Autodesk Fusion 360 part; units mm, degrees
note: some values were not read from the file. Set by a fixed rule: which sketch regions a step uses.
(part 4 of 6)
  line L2804 (355, -75.3453) -> (353, -74.1906)
  line L2805 (391.5, -47.1906) -> (389.5, -48.3453)
  line L2806 (378.5, -84.3453) -> (378.5, -86.6547)
  line L2807 (389.5, -75.3453) -> (389.5, -77.6547)
  line L2808 (384, -75.3453) -> (384, -77.6547)
  line L2809 (369.5, -74.1906) -> (367.5, -75.3453)
  line L2810 (390.75, -79.5822) -> (388.75, -78.4275)
  line L2811 (389.5, -48.3453) -> (389.5, -50.6547)
  line L2812 (369.5, -74.1906) -> (367.5, -75.3453)
  line L2813 (352.25, -88.5822) -> (350.25, -87.4275)
  line L2814 (386, -78.8094) -> (388, -77.6547)
  line L2815 (377.75, -83.0463) -> (379.75, -81.8916)
  line L2816 (364, -78.8094) -> (366, -77.6547)
  line L2817 (377, -77.6547) -> (377, -75.3453)
  line L2818 (366.75, -74.0463) -> (368.75, -72.8916)
  line L2819 (388.75, -51.4275) -> (386.75, -52.5822)
  line L2820 (389.5, -77.6547) -> (391.5, -78.8094)
  line L2821 (390.75, -52.5822) -> (388.75, -51.4275)
  line L2822 (368.75, -79.5822) -> (366.75, -78.4275)
  line L2823 (364.75, -72.8916) -> (366.75, -74.0463)
  line L2824 (389.5, -75.3453) -> (389.5, -77.6547)
  line L2825 (366, -75.3453) -> (364, -74.1906)
  line L2826 (371.5, -48.3453) -> (369.5, -47.1906)
  line L2827 (367.5, -75.3453) -> (367.5, -77.6547)
  line L2828 (346.75, -81.8916) -> (346.75, -79.5822)
  line L2829 (377.75, -78.4275) -> (375.75, -79.5822)
  line L2830 (388, -75.3453) -> (386, -74.1906)
  line L2831 (364, -78.8094) -> (366, -77.6547)
  line L2832 (345.5, -84.3453) -> (345.5, -86.6547)
  line L2833 (384, -57.3453) -> (384, -59.6547)
  line L2834 (390.75, -79.5822) -> (388.75, -78.4275)
  line L2835 (375.75, -79.5822) -> (375.75, -81.8916)
  line L2836 (384, -77.6547) -> (386, -78.8094)
  line L2837 (366, -77.6547) -> (366, -75.3453)
  line L2838 (348.25, -81.8916) -> (350.25, -83.0463)
  line L2839 (367.5, -57.3453) -> (367.5, -59.6547)
  line L2840 (379.75, -79.5822) -> (377.75, -78.4275)
  line L2841 (355.75, -56.0463) -> (357.75, -54.8916)
  line L2842 (348.25, -53.9293) -> (348.25, -54.8916)
  line L2843 (377.75, -47.0463) -> (379.75, -45.8916)
  line L2844 (384, -57.3453) -> (384, -59.6547)
  line L2845 (380.5, -74.1906) -> (378.5, -75.3453)
  line L2846 (349.5, -84.3453) -> (347.5, -83.1906)
  line L2847 (389.5, -57.3453) -> (389.5, -59.6547)
  line L2848 (380.5, -78.8094) -> (382.5, -77.6547)
  line L2849 (355, -59.6547) -> (355, -57.3453)
  line L2850 (381.25, -79.5822) -> (381.25, -81.8916)
  line L2851 (348.25, -79.5822) -> (348.25, -81.8916)
  line L2852 (391.5, -56.1906) -> (389.5, -57.3453)
  line L2853 (348.25, -79.5822) -> (348.25, -81.8916)
  line L2854 (368.75, -79.5822) -> (366.75, -78.4275)
  line L2855 (386.75, -43.5822) -> (386.75, -45.8916)
  line L2856 (367.5, -75.3453) -> (367.5, -77.6547)
  line L2857 (353, -83.1906) -> (351, -84.3453)
  line L2858 (380.5, -78.8094) -> (382.5, -77.6547)
  line L2859 (350.25, -87.4275) -> (348.25, -88.5822)
  line L2860 (386, -60.8094) -> (388, -59.6547)
  line L2861 (377.75, -78.4275) -> (375.75, -79.5822)
  line L2862 (357.75, -61.5822) -> (355.75, -60.4275)
  line L2863 (380.5, -51.8094) -> (382.5, -50.6547)
  line L2864 (378.5, -77.6547) -> (380.5, -78.8094)
  line L2865 (346.75, -81.8916) -> (346.75, -79.5822)
  line L2866 (388, -59.6547) -> (388, -57.3453)
  line L2867 (381.25, -79.5822) -> (381.25, -81.8916)
  line L2868 (375.75, -79.5822) -> (375.75, -81.8916)
  line L2869 (386, -56.1906) -> (384, -57.3453)
  line L2870 (367.5, -77.6547) -> (369.5, -78.8094)
  line L2871 (349.5, -84.3453) -> (347.5, -83.1906)
  line L2872 (364.75, -72.8916) -> (366.75, -74.0463)
  line L2873 (349.5, -86.6547) -> (349.5, -84.3453)
  line L2874 (380.5, -47.1906) -> (378.5, -48.3453)
  line L2875 (392.25, -61.5822) -> (392.25, -63.8916)
  line L2876 (390.75, -45.8916) -> (390.75, -45.244)
  line L2877 (357.75, -61.5822) -> (355.75, -60.4275)
  line L2878 (385.25, -45.8916) -> (385.25, -43.5822)
  line L2879 (366.75, -78.4275) -> (364.75, -79.5822)
  line L2880 (367.5, -77.6547) -> (369.5, -78.8094)
  line L2881 (382.5, -77.6547) -> (382.5, -75.3453)
  line L2882 (375.75, -43.5822) -> (375.75, -45.8916)
  line L2883 (353.75, -54.8916) -> (355.75, -56.0463)
  line L2884 (366, -75.3453) -> (364, -74.1906)
  line L2885 (346.75, -88.5822) -> (344.75, -87.4275)
  line L2886 (344.75, -83.0463) -> (346.75, -81.8916)
  line L2887 (356.5, -59.6547) -> (358.5, -60.8094)
  line L2888 (390.75, -45.8916) -> (390.75, -45.244)
  line L2889 (366, -59.6547) -> (366, -57.3453)
  line L2890 (382.5, -75.3453) -> (380.5, -74.1906)
  line L2891 (382.5, -75.3453) -> (380.5, -74.1906)
  line L2892 (386, -56.1906) -> (384, -57.3453)
  line L2893 (384, -59.6547) -> (386, -60.8094)
  line L2894 (351, -86.6547) -> (353, -87.8094)
  line L2895 (382.5, -50.6547) -> (382.5, -48.3453)
  line L2896 (358.5, -60.8094) -> (360.5, -59.6547)
  line L2897 (367.5, -57.3453) -> (367.5, -59.6547)
  line L2898 (379.75, -79.5822) -> (377.75, -78.4275)
  line L2899 (351, -84.3453) -> (351, -86.6547)
  line L2900 (355.75, -60.4275) -> (353.75, -61.5822)
  line L2901 (388.75, -60.4275) -> (386.75, -61.5822)
  line L2902 (352.25, -81.8916) -> (352.25, -79.5822)
  line L2903 (377, -77.6547) -> (377, -75.3453)
  arc A93 (390.75, -45.244) -> (386.8045, -43.5507) centre (375, -76.5) ccw
  line L2904 (386.8045, -43.5507) -> (386.75, -43.5822)
  line L2905 (351, -84.3453) -> (351, -86.6547)
  line L2906 (347.5, -83.1906) -> (345.5, -84.3453)
  line L2907 (349.5, -86.6547) -> (349.5, -84.3453)
  line L2908 (366, -59.6547) -> (366, -57.3453)
  line L2909 (377, -41.6547) -> (377, -41.5572)
  line L2910 (355.75, -60.4275) -> (353.75, -61.5822)
  line L2911 (345.5, -86.6547) -> (347.5, -87.8094)
  line L2912 (379.75, -81.8916) -> (379.75, -79.5822)
  line L2913 (351, -86.6547) -> (353, -87.8094)
  line L2914 (361.25, -60.4275) -> (359.25, -61.5822)
  line L2915 (385.25, -63.8916) -> (385.25, -61.5822)
  line L2916 (386.75, -54.8916) -> (388.75, -56.0463)
  line L2917 (344.75, -83.0463) -> (346.75, -81.8916)
  line L2918 (378.5, -50.6547) -> (380.5, -51.8094)
  line L2919 (378.5, -75.3453) -> (378.5, -77.6547)
  line L2920 (379.75, -52.5822) -> (377.75, -51.4275)
  line L2921 (359.25, -54.8916) -> (361.25, -56.0463)
  line L2922 (377.75, -47.0463) -> (379.75, -45.8916)
  line L2923 (367.5, -66.3453) -> (367.5, -68.6547)
  line L2924 (379.75, -81.8916) -> (379.75, -79.5822)
  line L2925 (352.25, -81.8916) -> (352.25, -79.5822)
  line L2926 (386.75, -54.8916) -> (388.75, -56.0463)
  line L2927 (386, -60.8094) -> (388, -59.6547)
  line L2928 (350.25, -83.0463) -> (352.25, -81.8916)
  line L2929 (360.5, -57.3453) -> (358.5, -56.1906)
  line L2930 (360.5, -57.3453) -> (358.5, -56.1906)
  line L2931 (378.5, -75.3453) -> (378.5, -77.6547)
  line L2932 (378.5, -48.3453) -> (378.5, -50.6547)
  line L2933 (378.5, -77.6547) -> (380.5, -78.8094)
  line L2934 (350.25, -87.4275) -> (348.25, -88.5822)
  line L2935 (355, -59.6547) -> (355, -57.3453)
  line L2936 (382.5, -50.6547) -> (382.5, -48.3453)
  line L2937 (391.5, -56.1906) -> (389.5, -57.3453)
  line L2938 (362, -57.3453) -> (362, -59.6547)
  line L2939 (388.75, -56.0463) -> (390.75, -54.8916)
  line L2940 (345.5, -86.6547) -> (347.5, -87.8094)
  line L2941 (379.75, -43.5822) -> (377.75, -42.4275)
  line L2942 (388.75, -60.4275) -> (386.75, -61.5822)
  line L2943 (347.5, -83.1906) -> (345.5, -84.3453)
  line L2944 (362, -57.3453) -> (362, -59.6547)
  line L2945 (377, -50.6547) -> (377, -48.3453)
  line L2946 (388, -57.3453) -> (386, -56.1906)
  line L2947 (381.25, -61.5822) -> (381.25, -63.8916)
  line L2948 (366, -66.3453) -> (364, -65.1906)
  line L2949 (382.5, -77.6547) -> (382.5, -75.3453)
  line L2950 (378.5, -48.3453) -> (378.5, -50.6547)
  line L2951 (388, -57.3453) -> (386, -56.1906)
  line L2952 (377, -50.6547) -> (377, -48.3453)
  line L2953 (358.5, -60.8094) -> (360.5, -59.6547)
  line L2954 (358.5, -56.1906) -> (356.5, -57.3453)
  line L2955 (389.5, -59.6547) -> (391.5, -60.8094)
  line L2956 (378.5, -50.6547) -> (380.5, -51.8094)
  line L2957 (382.5, -48.3453) -> (380.5, -47.1906)
  line L2958 (389.5, -59.6547) -> (391.5, -60.8094)
  line L2959 (350.25, -83.0463) -> (352.25, -81.8916)
  line L2960 (366.75, -69.4275) -> (364.75, -70.5822)
  line L2961 (358.5, -56.1906) -> (356.5, -57.3453)
  line L2962 (379.75, -52.5822) -> (377.75, -51.4275)
  line L2963 (388, -59.6547) -> (388, -57.3453)
  line L2964 (363.25, -63.8916) -> (363.25, -61.5822)
  line L2965 (351, -77.6547) -> (353, -78.8094)
  line L2966 (382.5, -48.3453) -> (380.5, -47.1906)
  line L2967 (359.25, -54.8916) -> (361.25, -56.0463)
  line L2968 (378.5436, -41.6798) -> (380.5, -42.8094)
  arc A94 (381.6602, -42.1395) -> (378.5436, -41.6798) centre (375, -76.5) ccw
  line L2969 (378.5436, -41.6798) -> (380.5, -42.8094)
  line L2970 (349.5, -77.6547) -> (349.5, -75.3453)
  line L2971 (377.75, -51.4275) -> (375.75, -52.5822)
  line L2972 (369.5, -56.1906) -> (367.5, -57.3453)
  line L2973 (380.5, -42.8094) -> (381.6602, -42.1395)
  line L2974 (375.75, -45.8916) -> (377.75, -47.0463)
  line L2975 (364.75, -54.8916) -> (366.75, -56.0463)
  line L2976 (367.5, -59.6547) -> (369.5, -60.8094)
  line L2977 (345.5, -84.3453) -> (345.5, -86.6547)
  line L2978 (347.5, -87.8094) -> (349.5, -86.6547)
  line L2979 (353.75, -54.8916) -> (355.75, -56.0463)
  line L2980 (375.75, -45.8916) -> (377.75, -47.0463)
  line L2981 (380.5, -47.1906) -> (378.5, -48.3453)
  line L2982 (353, -83.1906) -> (351, -84.3453)
  line L2983 (364, -60.8094) -> (366, -59.6547)
  line L2984 (356.5, -59.6547) -> (358.5, -60.8094)
  line L2985 (366.75, -51.4275) -> (364.75, -52.5822)
  line L2986 (368.75, -63.8916) -> (368.75, -61.5822)
  line L2987 (368.75, -63.8916) -> (368.75, -61.5822)
  line L2988 (366.75, -56.0463) -> (368.75, -54.8916)
  line L2989 (368.75, -61.5822) -> (366.75, -60.4275)
  line L2990 (353, -74.1906) -> (351, -75.3453)
  line L2991 (380.5, -51.8094) -> (382.5, -50.6547)
  line L2992 (360.5, -59.6547) -> (360.5, -57.3453)
  line L2993 (369.5, -65.1906) -> (367.5, -66.3453)
  line L2994 (348.25, -81.8916) -> (350.25, -83.0463)
  line L2995 (355.75, -56.0463) -> (357.75, -54.8916)
  line L2996 (390.75, -61.5822) -> (388.75, -60.4275)
  line L2997 (345.5, -75.3453) -> (345.5, -77.6547)
  line L2998 (367.5, -68.6547) -> (369.5, -69.8094)
  line L2999 (377.75, -42.4275) -> (375.75, -43.5822)
  line L3000 (368.75, -70.5822) -> (366.75, -69.4275)
  line L3001 (366, -57.3453) -> (364, -56.1906)
  line L3002 (390.75, -61.5822) -> (388.75, -60.4275)
  line L3003 (384, -59.6547) -> (386, -60.8094)
  line L3004 (346.75, -88.5822) -> (344.75, -87.4275)
  line L3005 (366.75, -56.0463) -> (368.75, -54.8916)
  line L3006 (350.25, -74.0463) -> (352.25, -72.8916)
  line L3007 (356.5, -57.3453) -> (356.5, -59.6547)
  arc A95 (383.427, -42.5296) -> (383.1782, -42.4689) centre (375, -76.5) ccw
  line L3008 (366, -66.3453) -> (364, -65.1906)
  line L3009 (377.75, -51.4275) -> (375.75, -52.5822)
  line L3010 (352.25, -79.5822) -> (350.25, -78.4275)
  line L3011 (345.5, -77.6547) -> (347.5, -78.8094)
  line L3012 (361.25, -60.4275) -> (359.25, -61.5822)
  line L3013 (352.25, -79.5822) -> (350.25, -78.4275)
  line L3014 (352.25, -88.5822) -> (350.25, -87.4275)
  line L3015 (369.5, -56.1906) -> (367.5, -57.3453)
  line L3016 (360.5, -59.6547) -> (360.5, -57.3453)
  line L3017 (388.75, -56.0463) -> (390.75, -54.8916)
  line L3018 (364.75, -70.5822) -> (364.75, -72.8916)
  line L3019 (385.25, -52.5822) -> (383.25, -51.4275)
  line L3020 (349.5, -77.6547) -> (349.5, -75.3453)
  line L3021 (364, -51.8094) -> (366, -50.6547)
  line L3022 (366.75, -65.0463) -> (368.75, -63.8916)
  line L3023 (347.5, -74.1906) -> (345.5, -75.3453)
  line L3024 (364.75, -52.5822) -> (364.75, -54.8916)
  line L3025 (379.75, -43.5822) -> (377.75, -42.4275)
  line L3026 (368.75, -54.8916) -> (368.75, -52.5822)
  line L3027 (380.5, -56.1906) -> (378.5, -57.3453)
  line L3028 (345.5, -75.3453) -> (345.5, -77.6547)
  line L3029 (367.5, -59.6547) -> (369.5, -60.8094)
  line L3030 (347.5, -74.1906) -> (345.5, -75.3453)
  line L3031 (385.25, -52.5822) -> (383.25, -51.4275)
  line L3032 (366, -57.3453) -> (364, -56.1906)
  line L3033 (381.25, -45.8916) -> (383.25, -47.0463)
  line L3034 (357.75, -54.8916) -> (357.75, -52.5822)
  line L3035 (357.75, -63.8916) -> (357.75, -61.5822)
  line L3036 (363.25, -54.8916) -> (363.25, -52.5822)
  line L3037 (383.1782, -42.4689) -> (381.25, -43.5822)
  line L3038 (383.25, -47.0463) -> (385.25, -45.8916)
  line L3039 (346.75, -79.5822) -> (344.75, -78.4275)
  line L3040 (383.25, -51.4275) -> (381.25, -52.5822)
  line L3041 (367.5, -50.6547) -> (369.5, -51.8094)
  line L3042 (351, -77.6547) -> (353, -78.8094)
  line L3043 (369.5, -65.1906) -> (367.5, -66.3453)
  line L3044 (366.75, -65.0463) -> (368.75, -63.8916)
  line L3045 (368.75, -52.5822) -> (366.75, -51.4275)
  line L3046 (380.5, -60.8094) -> (382.5, -59.6547)
  line L3047 (377.75, -42.4275) -> (375.75, -43.5822)
  line L3048 (367.5, -68.6547) -> (369.5, -69.8094)
  line L3049 (347.5, -78.8094) -> (349.5, -77.6547)
  arc A96 (390.75, -45.244) -> (386.8045, -43.5507) centre (375, -76.5) ccw
  line L3050 (344.75, -74.0463) -> (346.75, -72.8916)
  line L3051 (347.5, -78.8094) -> (349.5, -77.6547)
  line L3052 (363.25, -54.8916) -> (363.25, -52.5822)
  line L3053 (364.75, -63.8916) -> (366.75, -65.0463)
  line L3054 (359.25, -61.5822) -> (359.25, -63.8916)
  line L3055 (359.25, -61.5822) -> (359.25, -63.8916)
  line L3056 (350.25, -78.4275) -> (348.25, -79.5822)
  line L3057 (353.75, -61.5822) -> (353.75, -63.8916)
  line L3058 (385.25, -43.5822) -> (383.427, -42.5296)
  line L3059 (356.5, -57.3453) -> (356.5, -59.6547)
  line L3060 (377.75, -56.0463) -> (379.75, -54.8916)
  line L3061 (359.25, -52.5822) -> (359.25, -54.8916)
  line L3062 (383.25, -51.4275) -> (381.25, -52.5822)
  line L3063 (349.5, -75.3453) -> (347.5, -74.1906)
  line L3064 (363.25, -72.8916) -> (363.25, -70.5822)
  line L3065 (364.75, -61.5822) -> (364.75, -63.8916)
  line L3066 (350.25, -78.4275) -> (348.25, -79.5822)
  line L3067 (381.25, -61.5822) -> (381.25, -63.8916)
  line L3068 (364, -69.8094) -> (366, -68.6547)
  line L3069 (344.75, -74.0463) -> (346.75, -72.8916)
  line L3070 (366.75, -69.4275) -> (364.75, -70.5822)
  line L3071 (364.75, -52.5822) -> (364.75, -54.8916)
  line L3072 (377, -41.6547) -> (377, -41.5572)
  line L3073 (385.25, -43.5822) -> (383.427, -42.5296)
  line L3074 (383.1782, -42.4689) -> (381.25, -43.5822)
  line L3075 (367.5, -48.3453) -> (367.5, -50.6547)
  line L3076 (383.25, -47.0463) -> (385.25, -45.8916)
  line L3077 (353.75, -61.5822) -> (353.75, -63.8916)
  arc A97 (381.6602, -42.1395) -> (378.5436, -41.6798) centre (375, -76.5) ccw
  line L3078 (366.75, -51.4275) -> (364.75, -52.5822)
  line L3079 (381.25, -45.8916) -> (383.25, -47.0463)
  line L3080 (357.75, -63.8916) -> (357.75, -61.5822)
  line L3081 (366.75, -60.4275) -> (364.75, -61.5822)
  line L3082 (348.25, -72.8916) -> (350.25, -74.0463)
  line L3083 (386.8045, -43.5507) -> (386.75, -43.5822)
  line L3084 (368.75, -52.5822) -> (366.75, -51.4275)
  line L3085 (377, -59.6547) -> (377, -57.3453)
  line L3086 (368.75, -54.8916) -> (368.75, -52.5822)
  line L3087 (375.75, -54.8916) -> (377.75, -56.0463)
  line L3088 (346.75, -70.5822) -> (344.75, -69.4275)
  line L3089 (367.5, -48.3453) -> (367.5, -50.6547)
  line L3090 (364.75, -43.5822) -> (364.75, -45.8916)
  line L3091 (363.25, -63.8916) -> (363.25, -61.5822)
  line L3092 (350.25, -74.0463) -> (352.25, -72.8916)
  line L3093 (355, -57.3453) -> (353, -56.1906)
  line L3094 (377.75, -60.4275) -> (375.75, -61.5822)
  line L3095 (364.75, -54.8916) -> (366.75, -56.0463)
  line L3096 (355, -57.3453) -> (353, -56.1906)
  line L3097 (368.75, -72.8916) -> (368.75, -70.5822)
  line L3098 (390.75, -63.8916) -> (390.75, -61.5822)
  line L3099 (366, -50.6547) -> (366, -48.3453)
  line L3100 (378.5, -57.3453) -> (378.5, -59.6547)
  line L3101 (364.75, -61.5822) -> (364.75, -63.8916)
  line L3102 (348.25, -72.8916) -> (350.25, -74.0463)
  line L3103 (353, -74.1906) -> (351, -75.3453)
  line L3104 (353, -60.8094) -> (355, -59.6547)
  line L3105 (351, -75.3453) -> (351, -77.6547)
  line L3106 (355, -66.3453) -> (353, -65.1906)
  line L3107 (368.75, -70.5822) -> (366.75, -69.4275)
  line L3108 (351, -75.3453) -> (351, -77.6547)
  line L3109 (377.75, -60.4275) -> (375.75, -61.5822)
  line L3110 (345.5, -77.6547) -> (347.5, -78.8094)
  line L3111 (359.25, -45.244) -> (359.25, -45.8916)
  line L3112 (366, -68.6547) -> (366, -66.3453)
  line L3113 (380.5, -60.8094) -> (382.5, -59.6547)
  line L3114 (348.25, -63.8916) -> (350.25, -65.0463)
  line L3115 (359.25, -45.244) -> (359.25, -45.8916)
  line L3116 (377, -59.6547) -> (377, -57.3453)
  line L3117 (380.5, -42.8094) -> (381.6602, -42.1395)
  line L3118 (368.75, -45.8916) -> (368.75, -43.5822)
  line L3119 (382.5, -57.3453) -> (380.5, -56.1906)
  line L3120 (346.75, -79.5822) -> (344.75, -78.4275)
  line L3121 (383.25, -56.0463) -> (385.25, -54.8916)
  line L3122 (353, -69.8094) -> (355, -68.6547)
  line L3123 (377.75, -56.0463) -> (379.75, -54.8916)
  line L3124 (364, -60.8094) -> (366, -59.6547)
  line L3125 (382.5, -59.6547) -> (382.5, -57.3453)
  line L3126 (366, -50.6547) -> (366, -48.3453)
  line L3127 (366.75, -60.4275) -> (364.75, -61.5822)
  line L3128 (375.75, -61.5822) -> (375.75, -63.8916)
  line L3129 (364.75, -63.8916) -> (366.75, -65.0463)
  line L3130 (368.3398, -42.1395) -> (369.5, -42.8094)
  line L3131 (364, -51.8094) -> (366, -50.6547)
  line L3132 (368.75, -61.5822) -> (366.75, -60.4275)
  line L3133 (352.25, -70.5822) -> (350.25, -69.4275)
  line L3134 (386.75, -61.5822) -> (386.75, -63.8916)
  line L3135 (367.5, -66.3453) -> (367.5, -68.6547)
  line L3136 (367.5, -50.6547) -> (369.5, -51.8094)
  line L3137 (364, -69.8094) -> (366, -68.6547)
  line L3138 (353, -60.8094) -> (355, -59.6547)
  line L3139 (379.75, -61.5822) -> (377.75, -60.4275)
  line L3140 (366, -68.6547) -> (366, -66.3453)
  line L3141 (382.5, -59.6547) -> (382.5, -57.3453)
  line L3142 (349.5, -75.3453) -> (347.5, -74.1906)
  line L3143 (385.25, -63.8916) -> (385.25, -61.5822)
  line L3144 (363.25, -43.5822) -> (363.1955, -43.5507)
  line L3145 (356.5, -50.6547) -> (358.5, -51.8094)
  line L3146 (379.75, -61.5822) -> (377.75, -60.4275)
  line L3147 (363.25, -72.8916) -> (363.25, -70.5822)
  line L3148 (368.75, -72.8916) -> (368.75, -70.5822)
  arc A98 (350.4572, -51.5471) -> (348.25, -53.9293) centre (375, -76.5) ccw
  line L3149 (357.75, -52.5822) -> (355.75, -51.4275)
  line L3150 (351, -66.3453) -> (351, -68.6547)
  line L3151 (385.25, -61.5822) -> (383.25, -60.4275)
  line L3152 (382.5, -57.3453) -> (380.5, -56.1906)
  line L3153 (356.5, -48.3453) -> (356.5, -50.6547)
  line L3154 (378.5, -57.3453) -> (378.5, -59.6547)
  line L3155 (355, -48.3453) -> (354.558, -48.0901)
  line L3156 (364.75, -70.5822) -> (364.75, -72.8916)
  line L3157 (353, -65.1906) -> (351, -66.3453)
  line L3158 (361.25, -51.4275) -> (359.25, -52.5822)
  line L3159 (405.25, -83.0463) -> (407.25, -81.8916)
  line L3160 (409.917, -78.9084) -> (408.75, -79.5822)
  line L3161 (405.25, -78.4275) -> (403.25, -79.5822)
  line L3162 (403.25, -79.5822) -> (403.25, -81.8916)
  line L3163 (408, -78.8094) -> (409.9806, -77.6659)
  line L3164 (409.211, -83.8898) -> (408, -83.1906)
  line L3165 (407.25, -81.8916) -> (407.25, -79.5822)
  line L3166 (405.25, -78.4275) -> (403.25, -79.5822)
  line L3167 (407.25, -79.5822) -> (405.25, -78.4275)
  arc A99 (409.5109, -82.3309) -> (409.917, -78.9084) centre (375, -76.5) ccw
  line L3168 (408, -83.1906) -> (406, -84.3453)
  line L3169 (407.25, -79.5822) -> (405.25, -78.4275)
  line L3170 (408, -78.8094) -> (409.9806, -77.6659)
  line L3171 (407.25, -72.8916) -> (407.25, -70.5822)
  line L3172 (375, -51.8094) -> (377, -50.6547)
  line L3173 (407.25, -70.5822) -> (405.25, -69.4275)
  line L3174 (404.5, -77.6547) -> (404.5, -75.3453)
  line L3175 (405.25, -74.0463) -> (407.25, -72.8916)
  line L3176 (409.4268, -70.1914) -> (408.75, -70.5822)
  line L3177 (408, -74.1906) -> (406, -75.3453)
  line L3178 (403.25, -70.5822) -> (403.25, -72.8916)
  line L3179 (406, -68.6547) -> (408, -69.8094)
  arc A100 (409.8747, -73.5409) -> (409.4268, -70.1914) centre (375, -76.5) ccw
  line L3180 (405.25, -69.4275) -> (403.25, -70.5822)
  line L3181 (408.75, -70.5822) -> (408.75, -72.8916)
  line L3182 (407.25, -72.8916) -> (407.25, -70.5822)
  line L3183 (408.75, -72.8916) -> (409.8747, -73.5409)
  line L3184 (407.25, -70.5822) -> (405.25, -69.4275)
  line L3185 (405.25, -74.0463) -> (407.25, -72.8916)
  line L3186 (403.25, -70.5822) -> (403.25, -72.8916)
  line L3187 (408, -74.1906) -> (406, -75.3453)
  line L3188 (408.75, -70.5822) -> (408.75, -72.8916)
  line L3189 (403.25, -72.8916) -> (405.25, -74.0463)
  line L3190 (409.4268, -70.1914) -> (408.75, -70.5822)
  arc A101 (410, -76.5) -> (409.9806, -75.3341) centre (375, -76.5) ccw
  arc A102 (410, -76.5) -> (409.9806, -75.3341) centre (375, -76.5) ccw
  line L3191 (403.25, -72.8916) -> (405.25, -74.0463)
  line L3192 (409.9806, -75.3341) -> (408, -74.1906)
  line L3193 (409.9806, -75.3341) -> (408, -74.1906)
  line L3194 (408.75, -72.8916) -> (409.8747, -73.5409)
  line L3195 (405.25, -69.4275) -> (403.25, -70.5822)
  arc A103 (409.8747, -73.5409) -> (409.4268, -70.1914) centre (375, -76.5) ccw
  line L3196 (408, -69.8094) -> (409.211, -69.1102)
  line L3197 (406, -77.6547) -> (408, -78.8094)
  arc A104 (409.9806, -77.6659) -> (410, -76.5) centre (375, -76.5) ccw
  line L3198 (406, -77.6547) -> (408, -78.8094)
  line L3199 (406, -75.3453) -> (406, -77.6547)
  line L3200 (406, -68.6547) -> (408, -69.8094)
  line L3201 (406, -75.3453) -> (406, -77.6547)
  line L3202 (404.5, -77.6547) -> (404.5, -75.3453)
  line L3203 (408, -69.8094) -> (409.211, -69.1102)
  arc A105 (409.9806, -77.6659) -> (410, -76.5) centre (375, -76.5) ccw
  arc A106 (392.25, -106.9539) -> (394.4942, -105.5685) centre (375, -76.5) ccw
  line L3204 (394.4942, -105.5685) -> (394.25, -105.4275)
  line L3205 (394.25, -105.4275) -> (392.25, -106.5822)
  arc A107 (392.25, -106.9539) -> (394.4942, -105.5685) centre (375, -76.5) ccw
  line L3206 (394.25, -105.4275) -> (392.25, -106.5822)
  line L3207 (394.4942, -105.5685) -> (394.25, -105.4275)
  line L3208 (386.75, -99.8916) -> (388.75, -101.0463)
  line L3209 (399.5428, -51.5471) -> (397.75, -52.5822)
  line L3210 (381.25, -88.5822) -> (381.25, -90.8916)
  line L3211 (362, -77.6547) -> (364, -78.8094)
  line L3212 (396.25, -63.8916) -> (396.25, -61.5822)
  line L3213 (368.75, -81.8916) -> (368.75, -79.5822)
  line L3214 (371.5, -68.6547) -> (371.5, -66.3453)
  line L3215 (388, -95.6547) -> (388, -93.3453)
  line L3216 (399, -66.3453) -> (397, -65.1906)
  line L3217 (386, -96.8094) -> (388, -95.6547)
  line L3218 (397, -51.8094) -> (398.7552, -50.7961)
  arc A108 (398.7552, -50.7961) -> (395.442, -48.0901) centre (375, -76.5) ccw
  line L3219 (372.25, -96.4275) -> (370.25, -97.5822)
  line L3220 (386, -92.1906) -> (384, -93.3453)
  line L3221 (386.75, -99.8916) -> (388.75, -101.0463)
  line L3222 (372.25, -69.4275) -> (370.25, -70.5822)
  line L3223 (392.25, -97.5822) -> (392.25, -99.8916)
  line L3224 (399.5428, -51.5471) -> (397.75, -52.5822)
  line L3225 (393.5, -50.6547) -> (393.5, -48.3453)
  line L3226 (375, -101.1906) -> (373, -102.3453)
  line L3227 (372.25, -60.4275) -> (370.25, -61.5822)
  line L3228 (371.5, -68.6547) -> (371.5, -66.3453)
  line L3229 (374.25, -97.5822) -> (372.25, -96.4275)
  line L3230 (395.442, -48.0901) -> (395, -48.3453)
  line L3231 (395, -48.3453) -> (395, -50.6547)
  line L3232 (396.25, -63.8916) -> (396.25, -61.5822)
  line L3233 (389.5, -93.3453) -> (389.5, -95.6547)
  line L3234 (390.75, -97.5822) -> (388.75, -96.4275)
  line L3235 (401.75, -61.5822) -> (399.75, -60.4275)
  line L3236 (390.75, -54.8916) -> (390.75, -52.5822)
  line L3237 (395.442, -48.0901) -> (395, -48.3453)
  line L3238 (370.25, -63.8916) -> (372.25, -65.0463)
  line L3239 (392.25, -88.5822) -> (392.25, -90.8916)
  line L3240 (402.5, -60.8094) -> (404.5, -59.6547)
  line L3241 (370.25, -99.8916) -> (372.25, -101.0463)
  line L3242 (399, -66.3453) -> (397, -65.1906)
  line L3243 (395, -48.3453) -> (395, -50.6547)
  line L3244 (389.5, -95.6547) -> (391.5, -96.8094)
  line L3245 (372.25, -92.0463) -> (374.25, -90.8916)
  line L3246 (401.75, -61.5822) -> (399.75, -60.4275)
  line L3247 (353.75, -70.5822) -> (353.75, -72.8916)
  line L3248 (370.25, -97.5822) -> (370.25, -99.8916)
  line L3249 (396.25, -52.5822) -> (394.25, -51.4275)
  line L3250 (394.25, -65.0463) -> (396.25, -63.8916)
  line L3251 (372.25, -96.4275) -> (370.25, -97.5822)
  line L3252 (397.75, -63.8916) -> (399.75, -65.0463)
  line L3253 (395, -59.6547) -> (397, -60.8094)
  line L3254 (375, -92.1906) -> (373, -93.3453)
  line L3255 (404.1665, -57.1527) -> (402.5, -56.1906)
  line L3256 (373, -59.6547) -> (375, -60.8094)
  line L3257 (384, -95.6547) -> (386, -96.8094)
  line L3258 (375, -65.1906) -> (373, -66.3453)
  line L3259 (395, -50.6547) -> (397, -51.8094)
  line L3260 (363.25, -88.5822) -> (361.25, -87.4275)
  line L3261 (372.25, -65.0463) -> (374.25, -63.8916)
  line L3262 (397, -51.8094) -> (398.7552, -50.7961)
  line L3263 (395, -50.6547) -> (397, -51.8094)
  line L3264 (370.25, -63.8916) -> (372.25, -65.0463)
  line L3265 (397.75, -63.8916) -> (399.75, -65.0463)
  line L3266 (385.25, -90.8916) -> (385.25, -88.5822)
  line L3267 (370.25, -61.5822) -> (370.25, -63.8916)
  line L3268 (392.25, -97.5822) -> (392.25, -99.8916)
  line L3269 (397.75, -61.5822) -> (397.75, -63.8916)
  line L3270 (363.25, -52.5822) -> (361.25, -51.4275)
  line L3271 (360.5, -104.6547) -> (360.5, -102.3453)
  line L3272 (366.75, -87.4275) -> (364.75, -88.5822)
  line L3273 (359.25, -90.8916) -> (361.25, -92.0463)
  line L3274 (391.5, -51.8094) -> (393.5, -50.6547)
  line L3275 (342, -65.1906) -> (341.8476, -65.2786)
  line L3276 (395, -84.3453) -> (395, -86.6547)
  line L3277 (395, -84.3453) -> (395, -86.6547)
  line L3278 (406, -84.3453) -> (406, -86.6547)
  line L3279 (340.789, -69.1102) -> (342, -69.8094)
  line L3280 (372.25, -87.4275) -> (370.25, -88.5822)
  line L3281 (342, -65.1906) -> (341.8476, -65.2786)
  line L3282 (393.5, -86.6547) -> (393.5, -84.3453)
  line L3283 (342, -74.1906) -> (340.0194, -75.3341)
  line L3284 (359.25, -99.8916) -> (361.25, -101.0463)
  line L3285 (399, -86.6547) -> (399, -84.3453)
  line L3286 (364, -56.1906) -> (362, -57.3453)
  line L3287 (373, -84.3453) -> (373, -86.6547)
  arc A109 (341.8476, -65.2786) -> (340.789, -69.1102) centre (375, -76.5) ccw
  line L3288 (363.25, -61.5822) -> (361.25, -60.4275)
  line L3289 (341.25, -79.5822) -> (340.083, -78.9084)
  arc A110 (341.8476, -65.2786) -> (340.789, -69.1102) centre (375, -76.5) ccw
  line L3290 (361.25, -101.0463) -> (363.25, -99.8916)
  line L3291 (404.5, -86.6547) -> (404.5, -84.3453)
  line L3292 (361.25, -92.0463) -> (363.25, -90.8916)
  line L3293 (373, -84.3453) -> (373, -86.6547)
  line L3294 (394.25, -78.4275) -> (392.25, -79.5822)
  line L3295 (342, -78.8094) -> (344, -77.6547)
  line L3296 (400.5, -84.3453) -> (400.5, -86.6547)
  line L3297 (393.5, -57.3453) -> (391.5, -56.1906)
  arc A111 (340.789, -83.8898) -> (341.8476, -87.7214) centre (375, -76.5) ccw
  line L3298 (364.75, -106.5822) -> (364.75, -108.8916)
  line L3299 (362, -68.6547) -> (364, -69.8094)
  line L3300 (392.25, -81.8916) -> (394.25, -83.0463)
  line L3301 (368.75, -106.5822) -> (366.75, -105.4275)
  line L3302 (369.5, -87.8094) -> (371.5, -86.6547)
  line L3303 (356.5, -102.3453) -> (356.5, -104.6547)
  line L3304 (364.75, -108.8916) -> (366.75, -110.0463)
  line L3305 (393.5, -75.3453) -> (391.5, -74.1906)
  arc A112 (359.25, -107.756) -> (362.6388, -109.2445) centre (375, -76.5) ccw
  line L3306 (363.25, -97.5822) -> (361.25, -96.4275)
  line L3307 (344, -84.3453) -> (342, -83.1906)
  line L3308 (400.5, -84.3453) -> (400.5, -86.6547)
  line L3309 (341.25, -70.5822) -> (340.5732, -70.1914)
  line L3310 (394.25, -51.4275) -> (392.25, -52.5822)
  line L3311 (340.1253, -73.5409) -> (341.25, -72.8916)
  line L3312 (341.25, -81.8916) -> (341.25, -79.5822)
  line L3313 (393.5, -66.3453) -> (391.5, -65.1906)
  line L3314 (344, -75.3453) -> (342, -74.1906)
  line L3315 (364.75, -108.8916) -> (366.75, -110.0463)
  arc A113 (408.1524, -87.7214) -> (409.211, -83.8898) centre (375, -76.5) ccw
  line L3316 (344, -77.6547) -> (344, -75.3453)
  line L3317 (375, -83.1906) -> (373, -84.3453)
  line L3318 (363.25, -108.8916) -> (363.25, -106.5822)
  line L3319 (344, -77.6547) -> (344, -75.3453)
  line L3320 (364, -65.1906) -> (362, -66.3453)
  line L3321 (366.75, -105.4275) -> (364.75, -106.5822)
  line L3322 (363.25, -61.5822) -> (361.25, -60.4275)
  line L3323 (342.75, -79.5822) -> (342.75, -81.8916)
  line L3324 (399, -86.6547) -> (399, -84.3453)
  line L3325 (391.5, -87.8094) -> (393.5, -86.6547)
  line L3326 (344, -75.3453) -> (342, -74.1906)
  line L3327 (364.75, -81.8916) -> (366.75, -83.0463)
  line L3328 (406, -84.3453) -> (406, -86.6547)
  line L3329 (358.5, -105.8094) -> (360.5, -104.6547)
  line L3330 (373, -102.3453) -> (373, -104.6547)
  line L3331 (357.75, -106.9539) -> (357.75, -106.5822)
  line L3332 (364, -105.8094) -> (366, -104.6547)
  line L3333 (368.75, -106.5822) -> (366.75, -105.4275)
  line L3334 (355, -104.6547) -> (355, -102.3453)
  line L3335 (367.5, -84.3453) -> (367.5, -86.6547)
  line L3336 (361.25, -65.0463) -> (363.25, -63.8916)
  line L3337 (366, -86.6547) -> (366, -84.3453)
  line L3338 (363.25, -108.8916) -> (363.25, -106.5822)
  line L3339 (366.75, -83.0463) -> (368.75, -81.8916)
  line L3340 (392.25, -99.8916) -> (394.25, -101.0463)
  line L3341 (342.75, -79.5822) -> (342.75, -81.8916)
  line L3342 (355.75, -105.4275) -> (355.5058, -105.5685)
  line L3343 (354.558, -104.9099) -> (355, -104.6547)
  line L3344 (341.25, -79.5822) -> (340.083, -78.9084)
  line L3345 (391.5, -78.8094) -> (393.5, -77.6547)
  line L3346 (393.5, -66.3453) -> (391.5, -65.1906)
  line L3347 (366.75, -87.4275) -> (364.75, -88.5822)
  line L3348 (368.75, -108.8916) -> (368.75, -106.5822)
  line L3349 (366, -104.6547) -> (366, -102.3453)
  line L3350 (394.25, -96.4275) -> (392.25, -97.5822)
  line L3351 (340.1253, -73.5409) -> (341.25, -72.8916)
  line L3352 (393.5, -86.6547) -> (393.5, -84.3453)
  line L3353 (394.25, -60.4275) -> (392.25, -61.5822)
  line L3354 (362, -104.6547) -> (364, -105.8094)
  line L3355 (393.5, -57.3453) -> (391.5, -56.1906)
  line L3356 (355, -104.6547) -> (355, -102.3453)
  line L3357 (340.0194, -77.6659) -> (342, -78.8094)
  arc A114 (408.1524, -87.7214) -> (409.211, -83.8898) centre (375, -76.5) ccw
  line L3358 (367.5, -84.3453) -> (367.5, -86.6547)
  line L3359 (362, -86.6547) -> (364, -87.8094)
  line L3360 (356.5, -102.3453) -> (356.5, -104.6547)
  line L3361 (362.6388, -109.2445) -> (363.25, -108.8916)
  line L3362 (362, -102.3453) -> (362, -104.6547)
  line L3363 (368.75, -88.5822) -> (366.75, -87.4275)
  line L3364 (342, -78.8094) -> (344, -77.6547)
  line L3365 (361.25, -83.0463) -> (363.25, -81.8916)
  line L3366 (366, -104.6547) -> (366, -102.3453)
  line L3367 (341.25, -81.8916) -> (341.25, -79.5822)
  line L3368 (364.75, -81.8916) -> (366.75, -83.0463)
  line L3369 (364, -87.8094) -> (366, -86.6547)
  line L3370 (360.5, -104.6547) -> (360.5, -102.3453)
  line L3371 (342, -74.1906) -> (340.0194, -75.3341)
  line L3372 (340.0194, -77.6659) -> (342, -78.8094)
  line L3373 (357.75, -106.9539) -> (357.75, -106.5822)
  line L3374 (366, -84.3453) -> (364, -83.1906)
  line L3375 (363.25, -70.5822) -> (361.25, -69.4275)
  line L3376 (355.75, -105.4275) -> (355.5058, -105.5685)
  line L3377 (364, -105.8094) -> (366, -104.6547)
  arc A115 (340.0194, -75.3341) -> (340, -76.5) centre (375, -76.5) ccw
  line L3378 (353, -96.8094) -> (355, -95.6547)
  line L3379 (362, -104.6547) -> (364, -105.8094)
  line L3380 (362, -59.6547) -> (364, -60.8094)
  line L3381 (356.5, -104.6547) -> (358.5, -105.8094)
  arc A116 (340.0194, -75.3341) -> (340, -76.5) centre (375, -76.5) ccw
  line L3382 (356.5, -104.6547) -> (358.5, -105.8094)
  line L3383 (368.75, -88.5822) -> (366.75, -87.4275)
  line L3384 (355, -102.3453) -> (353, -101.1906)
  line L3385 (393.5, -68.6547) -> (393.5, -66.3453)
  line L3386 (392.25, -63.8916) -> (394.25, -65.0463)
  line L3387 (366.75, -105.4275) -> (364.75, -106.5822)
  arc A117 (404.5, -57.6652) -> (404.1665, -57.1527) centre (375, -76.5) ccw
  line L3388 (405.25, -60.4275) -> (403.25, -61.5822)
  line L3389 (399, -68.6547) -> (399, -66.3453)
  arc A118 (404.5, -57.6652) -> (404.1665, -57.1527) centre (375, -76.5) ccw
  line L3390 (357.75, -99.8916) -> (357.75, -97.5822)
  line L3391 (369.5, -83.1906) -> (367.5, -84.3453)
  line L3392 (355, -93.3453) -> (353, -92.1906)
  line L3393 (371.5, -104.6547) -> (371.5, -102.3453)
  line L3394 (359.25, -106.5822) -> (359.25, -107.756)
  arc A119 (368.3398, -110.8605) -> (371.4564, -111.3202) centre (375, -76.5) ccw
  arc A120 (409.211, -69.1102) -> (408.1524, -65.2786) centre (375, -76.5) ccw
  line L3395 (351, -93.3453) -> (351, -95.6547)
  line L3396 (369.5, -110.1906) -> (368.3398, -110.8605)
  line L3397 (369.5, -105.8094) -> (371.5, -104.6547)
  line L3398 (356.5, -93.3453) -> (356.5, -95.6547)
  line L3399 (407.25, -63.8916) -> (407.25, -62.9008)
  line L3400 (355, -102.3453) -> (353, -101.1906)
  line L3401 (364.75, -106.5822) -> (364.75, -108.8916)
  line L3402 (361.25, -47.0463) -> (363.25, -45.8916)
  line L3403 (371.4564, -111.3202) -> (369.5, -110.1906)
  line L3404 (400.5, -66.3453) -> (400.5, -68.6547)
  line L3405 (367.5, -104.6547) -> (369.5, -105.8094)
  line L3406 (392.25, -81.8916) -> (394.25, -83.0463)
  line L3407 (361.25, -56.0463) -> (363.25, -54.8916)
  line L3408 (356.5, -95.6547) -> (358.5, -96.8094)
  line L3409 (360.5, -95.6547) -> (360.5, -93.3453)
  line L3410 (350.25, -101.0463) -> (352.25, -99.8916)
  line L3411 (388.75, -74.0463) -> (390.75, -72.8916)
  line L3412 (357.75, -106.5822) -> (355.75, -105.4275)
  line L3413 (366.75, -83.0463) -> (368.75, -81.8916)
  line L3414 (364, -87.8094) -> (366, -86.6547)
  line L3415 (366.75, -110.0463) -> (368.75, -108.8916)
  line L3416 (400.5, -66.3453) -> (400.5, -68.6547)
  line L3417 (367.5, -86.6547) -> (369.5, -87.8094)
  line L3418 (399, -68.6547) -> (399, -66.3453)
  arc A121 (363.1955, -43.5507) -> (359.25, -45.244) centre (375, -76.5) ccw
  line L3419 (355, -93.3453) -> (353, -92.1906)
  line L3420 (366, -86.6547) -> (366, -84.3453)
  line L3421 (367.5, -86.6547) -> (369.5, -87.8094)
  line L3422 (369.5, -83.1906) -> (367.5, -84.3453)
  line L3423 (353, -96.8094) -> (355, -95.6547)
  line L3424 (358.5, -105.8094) -> (360.5, -104.6547)
  line L3425 (357.75, -106.5822) -> (355.75, -105.4275)
  line L3426 (366.75, -110.0463) -> (368.75, -108.8916)
  line L3427 (359.25, -106.5822) -> (359.25, -107.756)
  line L3428 (393.5, -68.6547) -> (393.5, -66.3453)
  line L3429 (367.5, -102.3453) -> (367.5, -104.6547)
  line L3430 (368.75, -108.8916) -> (368.75, -106.5822)
  line L3431 (354.558, -104.9099) -> (355, -104.6547)
  line L3432 (366, -84.3453) -> (364, -83.1906)
  line L3433 (362.6388, -109.2445) -> (363.25, -108.8916)
  line L3434 (351, -93.3453) -> (351, -95.6547)
  line L3435 (408, -65.1906) -> (406, -66.3453)
  line L3436 (371.4564, -111.3202) -> (369.5, -110.1906)
  line L3437 (360.5, -93.3453) -> (358.5, -92.1906)
  line L3438 (373, -102.3453) -> (373, -104.6547)
  line L3439 (377.75, -74.0463) -> (379.75, -72.8916)
  line L3440 (360.5, -102.3453) -> (358.5, -101.1906)
  arc A122 (348.25, -99.0707) -> (349.7943, -100.7831) centre (375, -76.5) ccw
  line L3441 (358.5, -96.8094) -> (360.5, -95.6547)
  line L3442 (353, -101.1906) -> (351.2448, -102.2039)
  line L3443 (388.75, -74.0463) -> (390.75, -72.8916)
  line L3444 (364, -83.1906) -> (362, -84.3453)
  line L3445 (355.75, -96.4275) -> (353.75, -97.5822)
  line L3446 (353, -92.1906) -> (351, -93.3453)
  line L3447 (404.5, -59.6547) -> (404.5, -57.6652)
  line L3448 (349.5, -95.6547) -> (349.5, -93.3453)
  line L3449 (369.5, -110.1906) -> (368.3398, -110.8605)
  line L3450 (353.75, -97.5822) -> (353.75, -99.8916)
  line L3451 (405.25, -60.4275) -> (403.25, -61.5822)
  line L3452 (353.75, -90.8916) -> (355.75, -92.0463)
  line L3453 (403.25, -61.5822) -> (403.25, -63.8916)
  line L3454 (355, -95.6547) -> (355, -93.3453)
  line L3455 (351, -95.6547) -> (353, -96.8094)
  line L3456 (360.5, -95.6547) -> (360.5, -93.3453)
  arc A123 (368.3398, -110.8605) -> (371.4564, -111.3202) centre (375, -76.5) ccw
  line L3457 (406.4359, -61.1121) -> (405.25, -60.4275)
  line L3458 (361.25, -74.0463) -> (363.25, -72.8916)
  line L3459 (406.4359, -61.1121) -> (405.25, -60.4275)
  line L3460 (357.75, -97.5822) -> (355.75, -96.4275)
  line L3461 (356.5, -93.3453) -> (356.5, -95.6547)
  line L3462 (353, -101.1906) -> (351.2448, -102.2039)
  line L3463 (363.25, -79.5822) -> (361.25, -78.4275)
  line L3464 (377.75, -74.0463) -> (379.75, -72.8916)
  line L3465 (352.25, -99.8916) -> (352.25, -97.5822)
  line L3466 (408.1524, -65.2786) -> (408, -65.1906)
  line L3467 (348.25, -97.5822) -> (348.25, -99.0707)
  line L3468 (356.5, -95.6547) -> (358.5, -96.8094)
  line L3469 (364, -47.1906) -> (362, -48.3453)
  line L3470 (358.5, -92.1906) -> (356.5, -93.3453)
  arc A124 (409.211, -69.1102) -> (408.1524, -65.2786) centre (375, -76.5) ccw
  arc A125 (363.1955, -43.5507) -> (359.25, -45.244) centre (375, -76.5) ccw
  line L3471 (371.5, -104.6547) -> (371.5, -102.3453)
  line L3472 (404.5, -59.6547) -> (404.5, -57.6652)
  line L3473 (369.5, -105.8094) -> (371.5, -104.6547)
  line L3474 (353.75, -99.8916) -> (355.75, -101.0463)
  line L3475 (367.5, -104.6547) -> (369.5, -105.8094)
  line L3476 (353, -92.1906) -> (351, -93.3453)
  line L3477 (353.75, -97.5822) -> (353.75, -99.8916)
  line L3478 (352.25, -99.8916) -> (352.25, -97.5822)
  line L3479 (355.75, -92.0463) -> (357.75, -90.8916)
  line L3480 (408.1524, -65.2786) -> (408, -65.1906)
  line L3481 (395, -66.3453) -> (395, -68.6547)
  line L3482 (350.25, -101.0463) -> (352.25, -99.8916)
  line L3483 (406, -66.3453) -> (406, -68.6547)
  arc A126 (348.25, -99.0707) -> (349.7943, -100.7831) centre (375, -76.5) ccw
  line L3484 (351, -95.6547) -> (353, -96.8094)
  line L3485 (348.25, -97.5822) -> (348.25, -99.0707)
  line L3486 (404.5, -68.6547) -> (404.5, -66.3453)
  line L3487 (374.25, -79.5822) -> (372.25, -78.4275)
  line L3488 (360.5, -93.3453) -> (358.5, -92.1906)
  arc A127 (407.25, -62.9008) -> (406.4359, -61.1121) centre (375, -76.5) ccw
  line L3489 (403.25, -63.8916) -> (405.25, -65.0463)
  line L3490 (364, -47.1906) -> (362, -48.3453)
  line L3491 (370.25, -72.8916) -> (372.25, -74.0463)
  line L3492 (403.25, -63.8916) -> (405.25, -65.0463)
  line L3493 (386.75, -72.8916) -> (388.75, -74.0463)
  line L3494 (373, -77.6547) -> (375, -78.8094)
  line L3495 (375.75, -72.8916) -> (377.75, -74.0463)
  line L3496 (388.75, -96.4275) -> (386.75, -97.5822)
  line L3497 (372.25, -74.0463) -> (374.25, -72.8916)
  line L3498 (362, -102.3453) -> (362, -104.6547)
  line L3499 (358.5, -101.1906) -> (356.5, -102.3453)
  line L3500 (373, -95.6547) -> (375, -96.8094)
  line L3501 (358.5, -96.8094) -> (360.5, -95.6547)
  line L3502 (371.5, -77.6547) -> (371.5, -75.3453)
  line L3503 (355, -95.6547) -> (355, -93.3453)
  line L3504 (388.75, -101.0463) -> (390.75, -99.8916)
  line L3505 (407.25, -63.8916) -> (407.25, -62.9008)
  line L3506 (375, -74.1906) -> (373, -75.3453)
  line L3507 (355.75, -92.0463) -> (357.75, -90.8916)
  line L3508 (367.5, -102.3453) -> (367.5, -104.6547)
  line L3509 (352.25, -97.5822) -> (350.25, -96.4275)
  line L3510 (359.25, -97.5822) -> (359.25, -99.8916)
  line L3511 (373, -75.3453) -> (373, -77.6547)
  line L3512 (406, -66.3453) -> (406, -68.6547)
  line L3513 (348.25, -90.8916) -> (350.25, -92.0463)
  line L3514 (404.5, -68.6547) -> (404.5, -66.3453)
  arc A128 (407.25, -62.9008) -> (406.4359, -61.1121) centre (375, -76.5) ccw
  line L3515 (371.5, -77.6547) -> (371.5, -75.3453)
  line L3516 (370.25, -90.8916) -> (372.25, -92.0463)
  line L3517 (388, -95.6547) -> (388, -93.3453)
  line L3518 (348.25, -90.8916) -> (350.25, -92.0463)
  line L3519 (355.75, -101.0463) -> (357.75, -99.8916)
  line L3520 (390.75, -97.5822) -> (388.75, -96.4275)
  line L3521 (405.25, -65.0463) -> (407.25, -63.8916)
  line L3522 (373, -75.3453) -> (373, -77.6547)
  line L3523 (349.7943, -100.7831) -> (350.25, -101.0463)
  line L3524 (372.25, -101.0463) -> (374.25, -99.8916)
  line L3525 (357.75, -99.8916) -> (357.75, -97.5822)
  line L3526 (350.25, -92.0463) -> (352.25, -90.8916)
  line L3527 (358.5, -101.1906) -> (356.5, -102.3453)
  line L3528 (383.25, -74.0463) -> (385.25, -72.8916)
  line L3529 (372.25, -78.4275) -> (370.25, -79.5822)
  line L3530 (362, -50.6547) -> (364, -51.8094)
  line L3531 (349.7943, -100.7831) -> (350.25, -101.0463)
  line L3532 (373, -77.6547) -> (375, -78.8094)
  line L3533 (353.75, -99.8916) -> (355.75, -101.0463)
  line L3534 (408, -65.1906) -> (406, -66.3453)
  line L3535 (390.75, -99.8916) -> (390.75, -97.5822)
  line L3536 (364, -65.1906) -> (362, -66.3453)
  line L3537 (350.25, -96.4275) -> (348.25, -97.5822)
  line L3538 (383.25, -74.0463) -> (385.25, -72.8916)
  line L3539 (372.25, -101.0463) -> (374.25, -99.8916)
  line L3540 (381.25, -72.8916) -> (383.25, -74.0463)
  line L3541 (360.5, -102.3453) -> (358.5, -101.1906)
  line L3542 (350.25, -92.0463) -> (352.25, -90.8916)
  line L3543 (385.25, -99.8916) -> (385.25, -97.5822)
  line L3544 (388.75, -92.0463) -> (390.75, -90.8916)
  line L3545 (352.25, -97.5822) -> (350.25, -96.4275)
  line L3546 (362, -68.6547) -> (364, -69.8094)
  line L3547 (385.25, -99.8916) -> (385.25, -97.5822)
  line L3548 (403.25, -61.5822) -> (403.25, -63.8916)
  line L3549 (405.25, -65.0463) -> (407.25, -63.8916)
  line L3550 (367.5, -95.6547) -> (369.5, -96.8094)
  line L3551 (353.75, -90.8916) -> (355.75, -92.0463)
  line L3552 (395, -66.3453) -> (395, -68.6547)
  line L3553 (357.75, -97.5822) -> (355.75, -96.4275)
  line L3554 (371.5, -95.6547) -> (371.5, -93.3453)
  line L3555 (370.25, -72.8916) -> (372.25, -74.0463)
  line L3556 (369.5, -101.1906) -> (367.5, -102.3453)
  line L3557 (369.5, -92.1906) -> (367.5, -93.3453)
  line L3558 (397.75, -52.5822) -> (397.75, -54.8916)
  line L3559 (397, -65.1906) -> (395, -66.3453)
  line L3560 (384, -95.6547) -> (386, -96.8094)
  line L3561 (374.25, -97.5822) -> (372.25, -96.4275)
  line L3562 (361.25, -74.0463) -> (363.25, -72.8916)
  line L3563 (388, -93.3453) -> (386, -92.1906)
  line L3564 (364, -56.1906) -> (362, -57.3453)
  line L3565 (374.25, -79.5822) -> (372.25, -78.4275)
  line L3566 (373, -95.6547) -> (375, -96.8094)
  line L3567 (369.5, -96.8094) -> (371.5, -95.6547)
  line L3568 (397, -60.8094) -> (399, -59.6547)
  line L3569 (388.75, -96.4275) -> (386.75, -97.5822)
  line L3570 (355.75, -101.0463) -> (357.75, -99.8916)
  line L3571 (372.25, -78.4275) -> (370.25, -79.5822)
  line L3572 (375, -101.1906) -> (373, -102.3453)
  line L3573 (373, -93.3453) -> (373, -95.6547)
  line L3574 (372.25, -92.0463) -> (374.25, -90.8916)
  line L3575 (371.5, -102.3453) -> (369.5, -101.1906)
  line L3576 (350.25, -96.4275) -> (348.25, -97.5822)
  line L3577 (359.25, -97.5822) -> (359.25, -99.8916)
  line L3578 (362, -50.6547) -> (364, -51.8094)
  line L3579 (375, -74.1906) -> (373, -75.3453)
  line L3580 (397.75, -52.5822) -> (397.75, -54.8916)
  line L3581 (384, -93.3453) -> (384, -95.6547)
  line L3582 (355.75, -96.4275) -> (353.75, -97.5822)
  line L3583 (367.5, -95.6547) -> (369.5, -96.8094)
  line L3584 (373, -93.3453) -> (373, -95.6547)
  line L3585 (372.25, -74.0463) -> (374.25, -72.8916)
  line L3586 (349.5, -95.6547) -> (349.5, -93.3453)
  line L3587 (369.5, -92.1906) -> (367.5, -93.3453)
  line L3588 (361.25, -65.0463) -> (363.25, -63.8916)
  arc A129 (401.75, -53.9293) -> (399.5428, -51.5471) centre (375, -76.5) ccw
  line L3589 (374.25, -99.8916) -> (374.25, -97.5822)
  line L3590 (369.5, -96.8094) -> (371.5, -95.6547)
  line L3591 (364, -74.1906) -> (362, -75.3453)
  arc A130 (401.75, -53.9293) -> (399.5428, -51.5471) centre (375, -76.5) ccw
  line L3592 (371.5, -102.3453) -> (369.5, -101.1906)
  line L3593 (381.25, -72.8916) -> (383.25, -74.0463)
  line L3594 (391.5, -92.1906) -> (389.5, -93.3453)
  line L3595 (388.75, -92.0463) -> (390.75, -90.8916)
  line L3596 (396.25, -54.8916) -> (396.25, -52.5822)
  line L3597 (371.5, -93.3453) -> (369.5, -92.1906)
  line L3598 (389.5, -95.6547) -> (391.5, -96.8094)
  line L3599 (375.75, -72.8916) -> (377.75, -74.0463)
  line L3600 (362, -77.6547) -> (364, -78.8094)
  line L3601 (370.25, -97.5822) -> (370.25, -99.8916)
  line L3602 (386.75, -97.5822) -> (386.75, -99.8916)
  line L3603 (362, -86.6547) -> (364, -87.8094)
  line L3604 (374.25, -99.8916) -> (374.25, -97.5822)
  line L3605 (390.75, -54.8916) -> (390.75, -52.5822)
  line L3606 (358.5, -92.1906) -> (356.5, -93.3453)
  line L3607 (370.25, -99.8916) -> (372.25, -101.0463)
  line L3608 (396.25, -54.8916) -> (396.25, -52.5822)
  line L3609 (384, -93.3453) -> (384, -95.6547)
  line L3610 (386.75, -72.8916) -> (388.75, -74.0463)
  line L3611 (363.25, -70.5822) -> (361.25, -69.4275)
  line L3612 (390.75, -99.8916) -> (390.75, -97.5822)
  line L3613 (370.25, -90.8916) -> (372.25, -92.0463)
  line L3614 (364, -83.1906) -> (362, -84.3453)
  line L3615 (396.25, -52.5822) -> (394.25, -51.4275)
  line L3616 (396.25, -61.5822) -> (394.25, -60.4275)
  line L3617 (371.5, -93.3453) -> (369.5, -92.1906)
  line L3618 (391.5, -92.1906) -> (389.5, -93.3453)
  line L3619 (386, -96.8094) -> (388, -95.6547)
  line L3620 (375, -92.1906) -> (373, -93.3453)
  line L3621 (373, -68.6547) -> (375, -69.8094)
  line L3622 (392.25, -52.5822) -> (392.25, -54.8916)
  line L3623 (371.5, -95.6547) -> (371.5, -93.3453)
  line L3624 (394.25, -65.0463) -> (396.25, -63.8916)
  line L3625 (400.5, -86.6547) -> (402.5, -87.8094)
  line L3626 (402.5, -96.8094) -> (404.1665, -95.8473)
  line L3627 (405.25, -83.0463) -> (407.25, -81.8916)
  line L3628 (403.25, -81.8916) -> (405.25, -83.0463)
  line L3629 (378.5, -102.3453) -> (378.5, -104.6547)
  line L3630 (388, -104.6547) -> (388, -102.3453)
  line L3631 (386, -105.8094) -> (388, -104.6547)
  line L3632 (377, -104.6547) -> (377, -102.3453)
  line L3633 (384, -102.3453) -> (384, -104.6547)
  line L3634 (378.5, -104.6547) -> (380.5, -105.8094)
  line L3635 (382.5, -104.6547) -> (382.5, -102.3453)
  line L3636 (385.25, -106.5822) -> (383.25, -105.4275)
  line L3637 (384, -104.6547) -> (386, -105.8094)
  line L3638 (383.25, -105.4275) -> (381.25, -106.5822)
  line L3639 (379.75, -106.5822) -> (377.75, -105.4275)
  line L3640 (377.75, -105.4275) -> (375.75, -106.5822)
  line L3641 (385.25, -106.5822) -> (383.25, -105.4275)
  line L3642 (378.5, -104.6547) -> (380.5, -105.8094)
  line L3643 (383.25, -105.4275) -> (381.25, -106.5822)
  line L3644 (382.5, -104.6547) -> (382.5, -102.3453)
  line L3645 (377, -104.6547) -> (377, -102.3453)
  line L3646 (378.5, -102.3453) -> (378.5, -104.6547)
  line L3647 (384, -102.3453) -> (384, -104.6547)
  line L3648 (377.75, -105.4275) -> (375.75, -106.5822)
  line L3649 (403.25, -81.8916) -> (405.25, -83.0463)
  arc A131 (409.5109, -82.3309) -> (409.917, -78.9084) centre (375, -76.5) ccw
  line L3650 (408.75, -81.8916) -> (409.5109, -82.3309)
  line L3651 (408.75, -79.5822) -> (408.75, -81.8916)
  line L3652 (409.917, -78.9084) -> (408.75, -79.5822)
  line L3653 (409.211, -83.8898) -> (408, -83.1906)
  line L3654 (407.25, -81.8916) -> (407.25, -79.5822)
  line L3655 (408.75, -81.8916) -> (409.5109, -82.3309)
  line L3656 (403.25, -79.5822) -> (403.25, -81.8916)
  line L3657 (408.75, -79.5822) -> (408.75, -81.8916)
  line L3658 (408, -83.1906) -> (406, -84.3453)
  arc A132 (378.5436, -111.3202) -> (381.6602, -110.8605) centre (375, -76.5) ccw
  line L3659 (386.75, -108.8916) -> (387.3612, -109.2445)
  line L3660 (386.75, -108.8916) -> (387.3612, -109.2445)
  line L3661 (375.75, -108.8916) -> (377.75, -110.0463)
  line L3662 (377.75, -110.0463) -> (379.75, -108.8916)
  line L3663 (383.25, -110.0463) -> (385.25, -108.8916)
  line L3664 (377, -111.4428) -> (377, -111.3453)
  line L3665 (383.25, -110.0463) -> (385.25, -108.8916)
  arc A133 (378.5436, -111.3202) -> (381.6602, -110.8605) centre (375, -76.5) ccw
  line L3666 (380.5, -110.1906) -> (378.5436, -111.3202)
  line L3667 (377, -111.4428) -> (377, -111.3453)
  line L3668 (381.6602, -110.8605) -> (380.5, -110.1906)
  line L3669 (380.5, -110.1906) -> (378.5436, -111.3202)
  line L3670 (377.75, -110.0463) -> (379.75, -108.8916)
  line L3671 (381.25, -108.8916) -> (383.25, -110.0463)
  line L3672 (375.75, -108.8916) -> (377.75, -110.0463)
  line L3673 (381.25, -108.8916) -> (383.25, -110.0463)
  line L3674 (381.6602, -110.8605) -> (380.5, -110.1906)
  line L3675 (353.75, -81.8916) -> (355.75, -83.0463)
  line L3676 (374.25, -70.5822) -> (372.25, -69.4275)
  line L3677 (388, -93.3453) -> (386, -92.1906)
  line L3678 (386, -92.1906) -> (384, -93.3453)
  line L3679 (399.75, -65.0463) -> (401.75, -63.8916)
  line L3680 (393.5, -50.6547) -> (393.5, -48.3453)
  line L3681 (374.25, -81.8916) -> (374.25, -79.5822)
  line L3682 (384, -68.6547) -> (386, -69.8094)
  line L3683 (402.5, -65.1906) -> (400.5, -66.3453)
  line L3684 (374.25, -63.8916) -> (374.25, -61.5822)
  line L3685 (363.25, -99.8916) -> (363.25, -97.5822)
  line L3686 (374.25, -63.8916) -> (374.25, -61.5822)
  line L3687 (369.5, -101.1906) -> (367.5, -102.3453)
  arc A134 (398.7552, -50.7961) -> (395.442, -48.0901) centre (375, -76.5) ccw
  line L3688 (370.25, -79.5822) -> (370.25, -81.8916)
  line L3689 (399.75, -60.4275) -> (397.75, -61.5822)